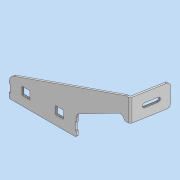
# Autodesk Inventor part: 0 零件
Saved by Autodesk Inventor 2020 (Build 240168000, 168)
## iProperties
Created: 2020-11-03
Part Number: 0 零件
Material: 一般
Document SubType Name: Modeling
Designer: p2013
Density: 1 g/cm^3
Appearance: 預設
Author: p2013
Autodesk Inventor part; units mm, degrees
ref_plane "YZ Plane" through (0, 0, 0) normal (1, 0, 0) x (0, 1, 0)
ref_plane "XZ Plane" through (0, 0, 0) normal (0, 1, 0) x (-1, 0, 0)
ref_plane "XY Plane" through (0, 0, 0) normal (0, 0, 1) x (1, 0, 0)
sketch "草圖1" plane through (0, 0, 0) normal (0, 0, 1) x (1, 0, 0)
  line L0 (0, 0) -> (-7.8042, 0) construction
  line L1 (0, 0) -> (0, -16.694) construction
  line L2 (0, 2) -> (0, 10.2)
  line L3 (230, 117.1064) -> (230, 74.1064)
  line L4 (130, 33.0474) -> (130, 10.2) construction
  line L5 (128, 0) -> (2, 0)
  line L6 (230, 117.1064) -> (288, 117.1064)
  line L7 (295, 110.1064) -> (295, 81.1064)
  line L8 (288, 74.1064) -> (230, 74.1064)
  line L9 (252, 99.6064) -> (274, 99.6064)
  arc A0 (274, 91.6064) -> (274, 99.6064) centre (274, 95.6064) ccw
  line L10 (274, 91.6064) -> (252, 91.6064)
  arc A1 (252, 99.6064) -> (252, 91.6064) centre (252, 95.6064) ccw
  line L11 (65, 14) -> (65, 14) construction
  arc A2 (10.0615, 42.1637) -> (0, 28) centre (15, 28) ccw
  line L12 (10.0615, 42.1637) -> (223.401, 116.5489)
  line L13 (226.6934, 117.1064) -> (230, 117.1064)
  line L14 (230, 74.1064) -> (225, 74.1064)
  line L15 (211.9999, 81.3311) -> (135.4256, 41.9398)
  arc A3 (295, 110.1064) -> (288, 117.1064) centre (288, 110.1064) ccw
  arc A4 (288, 74.1064) -> (295, 81.1064) centre (288, 81.1064) ccw
  arc A5 (222.0606, 76.5064) -> (225, 74.1064) centre (225, 77.1064) ccw
  arc A6 (222.0606, 76.5064) -> (211.9999, 81.3311) centre (215.202, 75.1064) ccw
  arc A7 (226.6934, 117.1064) -> (223.401, 116.5489) centre (226.6934, 107.1064) ccw
  arc A8 (135.4256, 41.9398) -> (130, 33.0474) centre (140, 33.0474) ccw
  line L16 (24.9, 33) -> (40.1, 33)
  line L17 (40.1, 33) -> (40.1, 18)
  line L18 (40.1, 18) -> (24.9, 18)
  line L19 (24.9, 18) -> (24.9, 33)
  line L20 (89.9, 33) -> (105.1, 33)
  line L21 (105.1, 33) -> (105.1, 18)
  line L22 (105.1, 18) -> (89.9, 18)
  line L23 (89.9, 18) -> (89.9, 33)
  line L24 (40.1, 25.5) -> (89.9, 25.5) construction
  line L25 (0, 25.2) -> (2, 25.2)
  line L26 (2, 25.2) -> (2, 10.2)
  line L27 (2, 10.2) -> (0, 10.2)
  line L28 (0, 10.2) -> (0, 25.2) construction
  line L29 (65, 0) -> (65, 25.5) construction
  line L30 (130, 25.2) -> (128, 25.2)
  line L31 (128, 25.2) -> (128, 10.2)
  line L32 (128, 10.2) -> (130, 10.2)
  line L33 (130, 10.2) -> (130, 33.0474) construction
  arc A9 (0, 2) -> (2, 0) centre (2, 2) ccw
  arc A10 (128, 0) -> (130, 2) centre (128, 2) ccw
  line L34 (0, 10.2) -> (0, 25.2) construction
  line L35 (0, 25.2) -> (0, 28)
  line L36 (130, 33.0474) -> (130, 25.2)
  line L37 (130, 10.2) -> (130, 2)
  point P0 (130, 0)
  point P1 (295, 117.1064)
  point P2 (295, 74.1064)
  point P3 (130, 39.1487)
  point P4 (225, 117.1064)
  point P5 (225, 74.1064)
  point P6 (225, 88.0185)
  point P7 (32.5, 33)
  point P8 (97.5, 33)
  point P9 (0, 10.2)
  point P10 (130, 28)
  point P11 (130, 19.7875)
  point P12 (130, 19.7875)
  dimension "d0" = 130
  dimension "d2" = 43
  dimension "d3" = 65
  dimension "d4" = 8
  dimension "d5" = 30
  dimension "d7" = 18
  dimension "d8" = 230
  dimension "d14" = 14
  dimension "d17" = 21.5
  dimension "d20" = 15
  dimension "d21" = 28
  dimension "d23" = 5
  dimension "d24" = 7
  dimension "d26" = 3
  dimension "d28" = 35
  dimension "d29" = 7
  dimension "d30" = 5
  dimension "d31" = 10
  dimension "d32" = 10
  dimension "d33" = 8
  dimension "d34" = 15.2
  dimension "d35" = 15.2
  dimension "d36" = 15
  dimension "d37" = 65
  dimension "d38" = 33
  dimension "d39" = 15
  dimension "d40" = 2
  dimension "d41" = 10.2
  dimension "d42" = 2
  dimension "d43" = 27.222
  constraints: 77 end point, 27 tangent, 23 point on circle, 16 parallel, 15 point on line, 11 centre point, 9 horizontal, 7 midpoint, 7 perpendicular, 5 symmetric about line, 5 vertical, 5 vertical alignment, 2 collinear, 2 equal radius, 1 coincident
  measures "d0" distance between parallel lines of L4 L2
  measures "d2" distance between parallel lines of L6 L8
  measures "d3" distance between parallel lines of L7 L3
  measures "d4" distance between parallel lines of L10 L9
  measures "d7" distance edge to line of A1 L3
  measures "d8" distance between parallel lines of L3 L2
  measures "d14" distance from line of L5 L11.start
  measures "d17" distance from line of L6 A0.centre
  measures "d20" radius of A2
  measures "d21" distance of L0.start L35.end
  measures "d23" distance of point (225, 117.106) L3.start
  measures "d24" radius of A3
  measures "d26" radius of A5
  measures "d28" distance edge to line of A6 L13
  measures "d29" radius of A6
  measures "d30" distance of L3.end L14.end
  measures "d31" radius of A7
  measures "d32" radius of A8
  measures "d33" angle of L15 L12
  measures "d34" distance between parallel lines of L17 L19
  measures "d35" distance between parallel lines of L21 L23
  measures "d36" distance between parallel lines of L16 L18
  measures "d37" distance of point (32.5, 33) point (97.5, 33)
  measures "d38" distance between parallel lines of L5 L16
  measures "d39" distance between parallel lines of L27 L25
  measures "d40" distance between parallel lines of L28 L26
  measures "d41" distance between parallel lines of L27 L5
  measures "d42" radius of A9
  measures "d43" angle of L5 L15
extrude "擠出1" add sketch "草圖1" along normal blind 3.5
bend part "折彎零件1" radius 0.5 angle 80 line through (230, 117.1064, 0) along (0, -1, 0) centre toward (0, 0, -1) moving side (1, 0, 0) both sides no
ref_plane "工作平面1" through (65, 2, 0) normal (-1, 0, 0) x (0, 0, 1)
